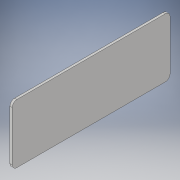
# Autodesk Inventor part: ZaslepkaObudowa
Saved by Autodesk Inventor 2019.4 (Build 234330000, 330)
## iProperties
Created: 2020-08-21
Part Number: ZaslepkaObudowa
Material: Ogólny
Document SubType Name: Konstrukcja blachowa
Designer: barto
Density: 1 g/cm^3
Sheet Metal Rule: Domyślny_mm
Appearance: Domyślna
Author: barto
Autodesk Inventor part; units mm, degrees
ref_plane "YZ Plane" through (0, 0, 0) normal (1, 0, 0) x (0, 1, 0)
ref_plane "XZ Plane" through (0, 0, 0) normal (0, 1, 0) x (-1, 0, 0)
ref_plane "XY Plane" through (0, 0, 0) normal (0, 0, 1) x (1, 0, 0)
sketch "Szkic1" plane through (0, 0, 0) normal (1, 0, 0) x (0, 1, 0)
  line L0 (-32.5, 103) -> (32.5, 103)
  line L1 (38.5, 97) -> (38.5, -97)
  line L2 (32.5, -103) -> (-32.5, -103)
  line L3 (-38.5, -97) -> (-38.5, 97)
  line L4 (-38.5, 103) -> (38.5, -103) construction
  arc A0 (32.5, -103) -> (38.5, -97) centre (32.5, -97) ccw
  arc A1 (-32.5, 103) -> (-38.5, 97) centre (-32.5, 97) ccw
  arc A2 (-38.5, -97) -> (-32.5, -103) centre (-32.5, -97) ccw
  arc A3 (38.5, 97) -> (32.5, 103) centre (32.5, 97) ccw
  point P0 (0, 0)
  dimension "d3" = 6
  measures "d3" radius of A0
extrude "Płyta1" add sketch "Szkic1" along normal blind 3
equation "\"d4\" = Grubość"
equation "\"PromieńGięcia\" = Grubość"
equation "\"SzerokośćGięciaPodcięcia\" = Grubość"
equation "\"GłębokośćGięciaPodcięcia\" = 0.5 * Grubość"
equation "\"RozmiarPodcięciaNarożnika\" = 4 * Grubość"
equation "\"MinimalnaPozostałość\" = 2 * Grubość"
equation "\"PromieńPrzejścia\" = PromieńGięcia"
equation "\"Rozmiar_promienia_Jacobiego\" = PromieńGięcia"
equation "\"Wielk_odstępu\" = Grubość"
equation "\"Grubość\" = 3"
